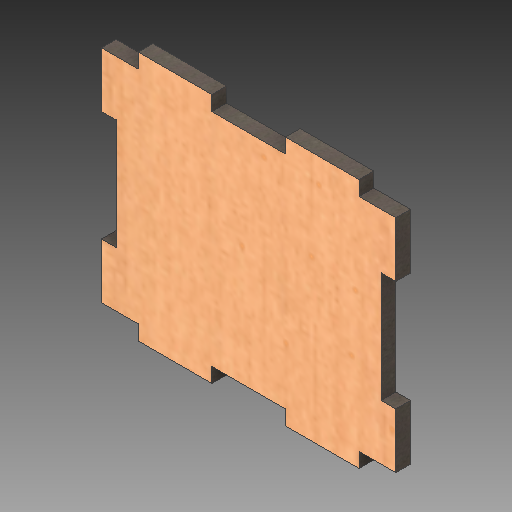
# Autodesk Inventor part: top
Saved by Autodesk Inventor 2019 (Build 230136000, 136)
## iProperties
Created: 2020-12-06
Part Number: top
Material: Дерево (береза)
Document SubType Name: Modeling
Designer: Professional
Density: 0.55 g/cm^3
Appearance: Береза — натуральный — полированный
Author: Professional
Autodesk Inventor part; units mm, degrees
ref_plane "YZ Plane" through (0, 0, 0) normal (1, 0, 0) x (0, 1, 0)
ref_plane "XZ Plane" through (0, 0, 0) normal (0, 1, 0) x (-1, 0, 0)
ref_plane "XY Plane" through (0, 0, 0) normal (0, 0, 1) x (1, 0, 0)
sketch "Эскиз1" plane through (0, 0, 0) normal (0, 0, 1) x (1, 0, 0)
  line L0 (0, 0) -> (-40, 0)
  line L1 (-40, -30) -> (-30, -30)
  line L2 (-30, -30) -> (-30, -34)
  line L3 (-30, -34) -> (-10, -34)
  line L4 (-10, -34) -> (-10, -30)
  line L5 (-10, -30) -> (0, -30)
  line L6 (-40, -30) -> (-40, -15)
  line L7 (-40, -15) -> (-36, -15)
  line L8 (-36, -15) -> (-36, 0)
  line L9 (-40, 30) -> (-30, 30)
  line L10 (-30, 30) -> (-30, 34)
  line L11 (-30, 34) -> (-10, 34)
  line L12 (-10, 34) -> (-10, 30)
  line L13 (-10, 30) -> (0, 30)
  line L14 (-40, 30) -> (-40, 15)
  line L15 (-40, 15) -> (-36, 15)
  line L16 (-36, 15) -> (-36, 0)
  line L17 (0, 30) -> (0, -30)
  line L18 (0, 0) -> (40, 0)
  line L19 (40, -30) -> (30, -30)
  line L20 (30, -30) -> (30, -34)
  line L21 (30, -34) -> (10, -34)
  line L22 (10, -34) -> (10, -30)
  line L23 (10, -30) -> (0, -30)
  line L24 (40, -30) -> (40, -15)
  line L25 (40, -15) -> (36, -15)
  line L26 (36, -15) -> (36, 0)
  line L27 (40, 30) -> (30, 30)
  line L28 (30, 30) -> (30, 34)
  line L29 (30, 34) -> (10, 34)
  line L30 (10, 34) -> (10, 30)
  line L31 (10, 30) -> (0, 30)
  line L32 (40, 30) -> (40, 15)
  line L33 (40, 15) -> (36, 15)
  line L34 (36, 15) -> (36, 0)
  dimension "d0" = 4
  dimension "d1" = 60
  dimension "d3" = 20
  dimension "d6" = 15
  dimension "d8" = 15
  dimension "d9" = 10
  dimension "d11" = 20
  constraints: 70 end point, 24 symmetric about line, 10 point on line, 6 perpendicular, 2 vertical, 1 horizontal, 1 midpoint
  measures "d0" distance of L1.end L2.end
  measures "d1" diameter of L1 L0
  measures "d3" distance between parallel lines of L4 L2
  measures "d6" distance of L7.end L8.end
  measures "d8" distance between parallel lines of L1 L7
  measures "d9" distance between parallel lines of L2 L6
  measures "d11" diameter of L4 L17
extrude "Выдавливание1" add sketch "Эскиз1" along normal blind 4
